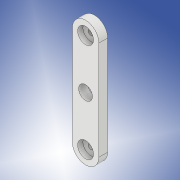
# Autodesk Inventor part: WaveGenerator
Saved by Autodesk Inventor 2017 SP1 (Build 210196100, 196)
## iProperties
Created: 2017-07-11
Part Number: WaveGenerator
Material: ABS Plastic
Document SubType Name: Modeling
Designer: zallen
Density: 1.06 g/cm^3
Appearance: CR White
Author: zallen
Autodesk Inventor part; units mm, degrees
ref_plane "YZ Plane" through (0, 0, 0) normal (1, 0, 0) x (0, 1, 0)
ref_plane "XZ Plane" through (0, 0, 0) normal (0, 1, 0) x (-1, 0, 0)
ref_plane "XY Plane" through (0, 0, 0) normal (0, 0, 1) x (1, 0, 0)
sketch "Sketch1" plane through (0, 0, 0) normal (0, 0, 1) x (1, 0, 0)
  line L0 (0, 0) -> (0, 71) construction
  circle A0 centre (0, 63.5) radius 7.5 construction
  circle A1 centre (0, 7.5) radius 7.5 construction
  line L1 (7.5, 63.5) -> (7.5, 7.5)
  line L2 (-7.5, 7.5) -> (-7.5, 63.5)
  arc A2 (7.5, 63.5) -> (-7.5, 63.5) centre (0, 63.5) ccw
  arc A3 (-7.5, 7.5) -> (7.5, 7.5) centre (0, 7.5) ccw
  circle A4 centre (0, 35.5) radius 3.9
  circle A5 centre (0, 63.5) radius 4.5
  circle A6 centre (0, 7.5) radius 4.5
  dimension "d1" = 15
  dimension "d2" = 15
  dimension "d3" = 7.8
  dimension "d4" = 9
  dimension "d5" = 9
  dimension "d25" = 56
  constraints: 10 point on circle, 7 centre point, 6 end point, 6 tangent, 2 coincident, 2 point on line, 1 concentric, 1 midpoint, 1 vertical
  measures "d1" diameter of A0
  measures "d2" diameter of A1
  measures "d3" diameter of A4
  measures "d4" diameter of A5
  measures "d5" diameter of A6
  measures "d25" distance of A1.centre A0.centre
extrude "Extrusion1" add sketch "Sketch1" along normal blind 3
sketch "Sketch7" plane through (0, 0, 0) normal (0, 0, -1) x (-1, 0, 0)
  circle A0 centre (0, 35.5) radius 3.9 projected
  circle A1 centre (0, 7.5) radius 4.5 projected
  circle A2 centre (0, 63.5) radius 4.5 projected
  line L0 (-7.5, 63.5) -> (-7.5, 7.5) projected
  arc A3 (-7.5, 7.5) -> (7.5, 7.5) centre (0, 7.5) ccw projected
  line L1 (7.5, 7.5) -> (7.5, 63.5) projected
  arc A4 (7.5, 63.5) -> (-7.5, 63.5) centre (0, 63.5) ccw projected
  circle A5 centre (0, 63.5) radius 1.5
  circle A6 centre (0, 7.5) radius 1.5
  point P0 (0, 0)
  dimension "d21" = 3
  dimension "d22" = 3
  constraints: 2 centre point, 2 coincident
  measures "d21" diameter of A5
  measures "d22" diameter of A6
extrude "Extrusion6" add sketch "Sketch7" along normal blind 2 contours A1 | A2 | A4 L1 A3 L0
body "Solid1"
